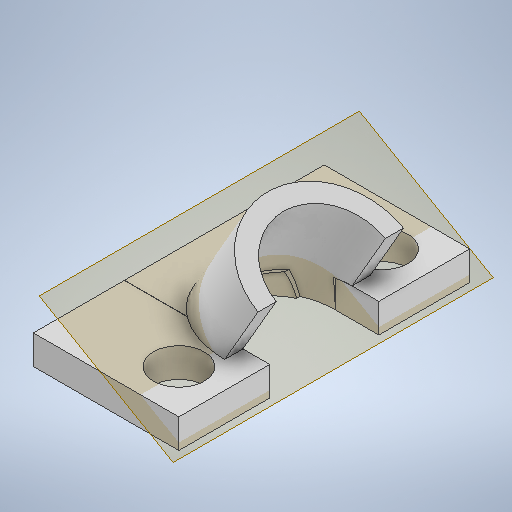
# Autodesk Inventor part: Front Bracket
Saved by Autodesk Inventor 2026.2 (Build 302298010, 298A)
## iProperties
Created: 2026-05-02
Part Number: Front Bracket
Material: Generic
Document SubType Name: Modeling
Designer: piete
Density: 1 g/cm^3
Appearance: Default
Author: piete
Autodesk Inventor part; units mm, degrees
ref_plane "YZ Plane" through (0, 0, 0) normal (1, 0, 0) x (0, 1, 0)
ref_plane "XZ Plane" through (0, 0, 0) normal (0, 1, 0) x (-1, 0, 0)
ref_plane "XY Plane" through (0, 0, 0) normal (0, 0, 1) x (1, 0, 0)
sketch "Sketch1" plane through (0, 0, 0) normal (0, 1, 0) x (-1, 0, 0)
  circle A0 centre (0, 7) radius 1.75
  circle A1 centre (0, -7) radius 1.75
  line L0 (7, 10) -> (-3, 10)
  line L1 (-3, 10) -> (-3, -10)
  line L2 (-3, -10) -> (7, -10)
  line L3 (7, -10) -> (7, 10)
  line L4 (7, 3.75) -> (-0.3, 3.75)
  line L5 (-0.3, 3.75) -> (-0.3, -3.75)
  line L6 (-0.3, -3.75) -> (7, -3.75)
  line L7 (7, -3.75) -> (7, 3.75)
  point P0 (0, 0)
  dimension "d0" = 3.5
  dimension "d1" = 3.5
  dimension "d2" = 0
  dimension "d3" = 0
  dimension "d4" = 14
  dimension "d5" = 7
  dimension "d6" = 3
  dimension "d7" = 3
  dimension "d8" = 3
  dimension "d9" = 10
  dimension "d10" = 7.5
  dimension "d11" = 3.75
  dimension "d12" = 0.3
  constraints: 16 end point, 4 parallel, 2 centre point, 2 horizontal, 2 perpendicular, 1 point on line
  measures "d0" diameter of A0
  measures "d1" diameter of A1
  measures "d2" horizontal distance of A0.centre A1.centre
  measures "d3" horizontal distance of point (0, 0) A0.centre
  measures "d4" distance of A1.centre A0.centre
  measures "d5" distance of point (0, 0) A0.centre
  measures "d6" distance from line of L1 A1.centre
  measures "d7" distance from line of A1.centre L2
  measures "d8" distance from line of L0 A0.centre
  measures "d9" distance between parallel lines of L1 L3
  measures "d10" distance of L5.end L4.end
  measures "d11" distance from line of L4 point (0, 0)
  measures "d12" distance from line of point (0, 0) L5
extrude "Extrusion1" add sketch "Sketch1" along normal blind 2 contours L3 L4 L5 L6 L2 L1 L0
ref_plane "Work Plane1" through (0.3, 2, -3.75) normal (0.5, 0.866, 0) x (0, 0, 1)
sketch "Sketch2" plane through (0.3, 2, -3.75) normal (0.5, 0.866, 0) x (0, 0, 1)
  line L0 (0, 0) -> (7.5, 0) projected
  circle A0 centre (3.75, 0) radius 3.75
  point P0 (3.75, 0.7402)
  dimension "d16" = 7.5
  constraints: 1 centre point, 1 midpoint
  measures "d16" diameter of A0
extrude "Extrusion2" cut sketch "Sketch2" along normal through all both and the other way through all
sketch "Sketch3" plane through (0.3, 2, -3.75) normal (0.5, 0.866, 0) x (0, 0, 1)
  circle A0 centre (3.75, 0.7402) radius 3.75
  circle A1 centre (3.75, 0.7402) radius 5
  line L0 (8.75, 0.7402) -> (-1.25, 0.7402)
  point P0 (7.5, 0.7402)
  point P1 (0, 0.7402)
  dimension "d19" = 7.5
  dimension "d20" = 10
  constraints: 2 centre point, 2 coincident, 2 end point, 2 point on circle
  measures "d19" diameter of A0
  measures "d20" diameter of A1
extrude "Extrusion3" add sketch "Sketch3" along normal mid plane 10 contours L0 A1 A0 picked at (8.2486, 0.0422)
sketch "Sketch4" plane through (-7, 0, -10) normal (-1, 0, 0) x (0, 0, 1)
  line L0 (6.25, 0) -> (5, 0) projected
  line L1 (12.9317, 2) -> (13.7317, 2) projected
  line L2 (6.25, 0) -> (13.7317, 0)
  line L3 (13.7317, 0) -> (13.7317, 2)
  line L4 (13.7317, 2) -> (6.25, 2)
  line L5 (6.25, 2) -> (6.25, 0)
  point P0 (10, 0)
  point P1 (12.9317, 2)
  constraints: 8 end point, 2 parallel, 1 horizontal, 1 perpendicular
extrude "Extrusion4" add sketch "Sketch4" against normal blind 5
sketch "Sketch5" plane through (-7, 0, 10) normal (0, 0, 1) x (1, 0, 0)
  line L0 (0, 0) -> (0, 2) projected
  line L1 (0, 0) -> (10, 0)
  line L2 (10, 0) -> (10, -5)
  line L3 (10, -5) -> (0, -5)
  line L4 (0, -5) -> (0, 0)
  point P0 (7, 0)
  dimension "d25" = 10
  dimension "d26" = 5
  constraints: 8 end point, 2 parallel, 1 horizontal, 1 perpendicular
  measures "d25" distance of L2.end L3.end
  measures "d26" distance of L1.end L2.end
extrude "Extrusion5" cut sketch "Sketch5" against normal through all
sketch "Sketch6" plane through (0.3, 2, -3.75) normal (0.5, 0.866, 0) x (0, 0, 1)
  circle A0 centre (3.75, 0.7402) radius 3.55
  dimension "d29" = 7.1
  constraints: 1 centre point, 1 coincident
  measures "d29" diameter of A0
extrude "Extrusion6" cut sketch "Sketch6" against normal through all
sketch "Sketch7" plane through (0, 0, 0) normal (0, -1, 0) x (1, 0, 0)
  ellipse E0 centre (0, 0) end of major axis (-4.3301, 0) minor radius 3.75 (0, 3.75) -> (0, -3.75) ccw projected
  line L0 (3, -2.9317) -> (3, -10) projected
  line L1 (0, 3.75) -> (3, 3.75)
  line L2 (3, 3.75) -> (3, -3.75)
  line L3 (3, -3.75) -> (0, -3.75)
  line L4 (0, -3.75) -> (0, 3.75)
  point P0 (0, 0)
  dimension "d32" = 7.5
  constraints: 8 end point, 2 parallel, 1 horizontal, 1 perpendicular, 1 point on line, 1 other
  measures "d32" distance of L1.end L2.end
extrude "Extrusion7" cut sketch "Sketch7" against normal up to surface (2 mm away) contours L1 L2 L0 L3 L4
equation "\"d11\" = 0.5 * d10"
body "Solid1"
